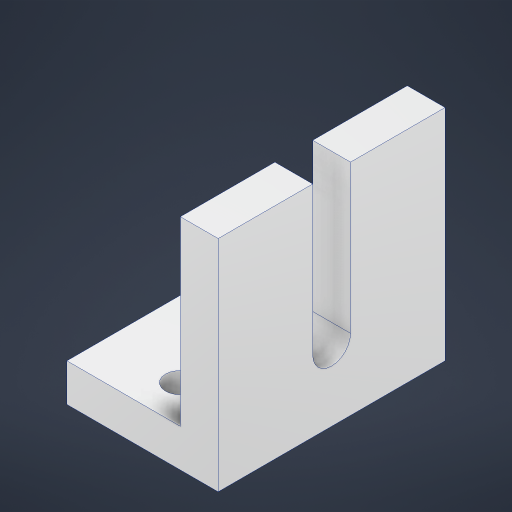
# Autodesk Inventor part: BUMPER BRACKETS
Saved by Autodesk Inventor 2024.3 (Build 283343000, 343)
## iProperties
Created: 2024-12-08
Part Number: BUMPER BRACKETS
Material: Aluminum 6061
Document SubType Name: Modeling
Designer: kaito
Density: 2.7 g/cm^3
Appearance: Aluminum - Flat
Author: kaito
Autodesk Inventor part; units mm, degrees
ref_plane "YZ Plane" through (0, 0, 0) normal (1, 0, 0) x (0, 1, 0)
ref_plane "XZ Plane" through (0, 0, 0) normal (0, 1, 0) x (-1, 0, 0)
ref_plane "XY Plane" through (0, 0, 0) normal (0, 0, 1) x (1, 0, 0)
sketch "Sketch1" plane through (0, 0, 0) normal (0, 1, 0) x (-1, 0, 0)
  line L0 (0, 0) -> (25.4, 0)
  line L1 (25.4, 0) -> (25.4, -38.1)
  line L2 (25.4, -38.1) -> (0, -38.1)
  line L3 (0, -38.1) -> (0, 0)
  circle A0 centre (12.7, -6.35) radius 2.4892
  circle A1 centre (12.7, -19.05) radius 2.4892
  circle A2 centre (12.7, -31.75) radius 2.4892
  point P0 (12.7, -38.1)
  dimension "d1" = 38.1
  dimension "d2" = 25.4
  dimension "d3" = 4.9784
  dimension "d4" = 6.35
  dimension "d7" = 12.7
  constraints: 8 end point, 3 centre point, 2 parallel, 1 horizontal, 1 midpoint, 1 perpendicular, 1 vertical, 1 vertical alignment, 4 other
  measures "d1" distance of L2.end L0.start
  measures "d2" distance of L1.end L2.end
  measures "d3" diameter of A0
  measures "d4" distance from line of L0 A0.centre
  measures "d7" distance of A0.centre A1.centre
extrude "Extrusion1" add sketch "Sketch1" along normal blind 6.35
sketch "Sketch2" plane through (0, 6.35, 0) normal (0, 1, 0) x (1, 0, 0)
  line L0 (0, 38.1) -> (-25.4, 38.1) projected
  line L1 (0, 38.1) -> (-6.35, 38.1)
  line L2 (-6.35, 38.1) -> (-6.35, 0)
  line L3 (-6.35, 0) -> (0, 0)
  line L4 (0, 0) -> (0, 38.1)
  point P0 (0, 0)
  dimension "d14" = 6.35
  dimension "d15" = 38.1
  constraints: 8 end point, 2 parallel, 1 horizontal, 1 perpendicular
  measures "d14" distance of L3.end L2.end
  measures "d15" distance of L3.end L0.start
extrude "Extrusion2" add sketch "Sketch2" along normal blind 30.48
sketch "Sketch3" plane through (0, 0, 0) normal (1, 0, 0) x (0, 0, -1)
  line L0 (0, 6.35) -> (0, 36.83) projected
  line L1 (0, 36.83) -> (15.875, 36.8288)
  line L2 (38.1, 6.35) -> (38.1, 36.83) projected
  line L3 (38.1, 36.83) -> (22.225, 36.83)
  line L4 (38.1, 36.83) -> (0, 36.83) projected
  line L5 (22.225, 36.83) -> (15.8731, 36.83)
  line L6 (15.8731, 36.83) -> (15.8731, 11.9339)
  line L7 (22.225, 11.9339) -> (22.225, 36.83)
  arc A0 (15.8731, 11.9339) -> (22.225, 11.9339) centre (19.049, 11.9339) ccw
  point P0 (0, 0)
  dimension "d18" = 15.875
  dimension "d19" = 15.875
  constraints: 10 end point, 2 point on circle, 1 centre point, 1 horizontal, 1 parallel, 1 perpendicular, 1 point on line, 1 tangent
  measures "d18" distance of L0.end L1.end
  measures "d19" distance of L2.end L3.end
extrude "Extrusion3" cut sketch "Sketch3" against normal blind 30.48
body "Solid1"
